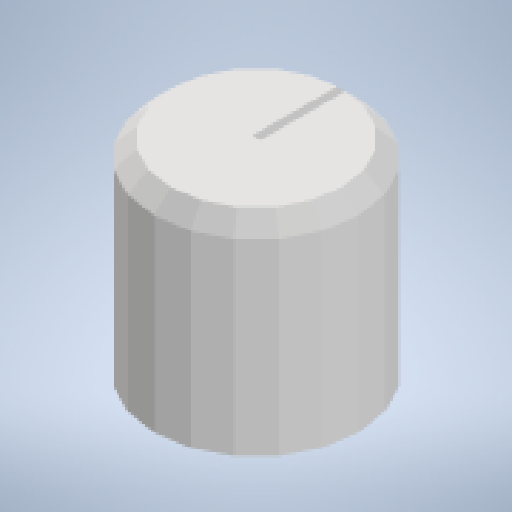
# Autodesk Inventor part: PotiBoxKnob
Saved by Autodesk Inventor 2024.3 (Build 283343000, 343)
## iProperties
Created: 2025-03-30
Part Number: PotiBoxKnob
Material: Generisch
Document SubType Name: Modeling
Designer: maxho
Density: 1 g/cm^3
Appearance: Vorgabe
Author: maxho
## iProperties of the stored document PotiBoxKnob_3D-Druck.ipt
Created: 2025-03-30
Part Number: PotiBoxKnob_3D-Druck
Material: Generisch
Document SubType Name: Modeling
Designer: maxho
Density: 1 g/cm^3
Appearance: Vorgabe
Author: maxho
Autodesk Inventor part; units mm, degrees
ref_plane "YZ Plane" through (0, 0, 0) normal (1, 0, 0) x (0, 1, 0)
ref_plane "XZ Plane" through (0, 0, 0) normal (0, 1, 0) x (-1, 0, 0)
ref_plane "XY Plane" through (0, 0, 0) normal (0, 0, 1) x (1, 0, 0)
sketch "Skizze1" plane through (0, 0, 0) normal (0, 0, 1) x (1, 0, 0)
  circle A0 centre (0, 0) radius 12.5 construction
  line L0 (-0.5, 16.5) -> (0.5, 16.5)
  line L1 (0.5, 16.5) -> (0.5, 11.5)
  line L2 (0.5, 11.5) -> (-0.5, 11.5)
  line L3 (-0.5, 11.5) -> (-0.5, 16.5)
  line L4 (0, -12.5) -> (-3.8627, -11.8882)
  line L5 (-3.8627, -11.8882) -> (-7.3473, -10.1127)
  line L6 (-7.3473, -10.1127) -> (-10.1127, -7.3473)
  line L7 (-10.1127, -7.3473) -> (-11.8882, -3.8627)
  line L8 (-11.8882, -3.8627) -> (-12.5, 0)
  line L9 (-12.5, 0) -> (-11.8882, 3.8627)
  line L10 (-11.8882, 3.8627) -> (-10.1127, 7.3473)
  line L11 (-10.1127, 7.3473) -> (-7.3473, 10.1127)
  line L12 (-7.3473, 10.1127) -> (-3.8627, 11.8882)
  line L13 (-3.8627, 11.8882) -> (0, 12.5)
  line L14 (0, 12.5) -> (3.8627, 11.8882)
  line L15 (3.8627, 11.8882) -> (7.3473, 10.1127)
  line L16 (7.3473, 10.1127) -> (10.1127, 7.3473)
  line L17 (10.1127, 7.3473) -> (11.8882, 3.8627)
  line L18 (11.8882, 3.8627) -> (12.5, 0)
  line L19 (12.5, 0) -> (11.8882, -3.8627)
  line L20 (11.8882, -3.8627) -> (10.1127, -7.3473)
  line L21 (10.1127, -7.3473) -> (7.3473, -10.1127)
  line L22 (7.3473, -10.1127) -> (3.8627, -11.8882)
  line L23 (3.8627, -11.8882) -> (0, -12.5)
  point P0 (0, 11.5)
  point P1 (-0.5, 12.49)
  point P2 (0.5, 12.49)
  point P3 (-0.5, 12.4208)
  point P4 (0.5, 12.4208)
  dimension "d0" = 25
  dimension "d3" = 1
  dimension "d4" = 1
  dimension "d12" = 5
  constraints: 48 end point, 2 coincident, 2 parallel, 2 vertical alignment, 1 horizontal, 1 midpoint, 1 perpendicular, 44 other
  measures "d3" length of L2
  measures "d4" distance of L0.start L0.end
  measures "d12" distance between parallel lines of L0 L2
extrude "Extrusion1" add sketch "Skizze1" along normal blind 25 contours L3 L2 L1 L14 L15 L16 L17 L18 L19 L20 L21 L22 L23 L4 L5 L6 L7 L8 L9 L10 L11 L12 L13
sketch "Skizze4" plane through (0, 0, 25) normal (0, 0, 1) x (1, 0, 0)
  line L0 (-0.5, 11.5) -> (-0.5, 12.4208) projected
  line L1 (-0.5, 12.4208) -> (-3.8627, 11.8882) projected
  line L2 (-3.8627, 11.8882) -> (-7.3473, 10.1127) projected
  line L3 (-7.3473, 10.1127) -> (-10.1127, 7.3473) projected
  line L4 (-10.1127, 7.3473) -> (-11.8882, 3.8627) projected
  line L5 (-11.8882, 3.8627) -> (-12.5, 0) projected
  line L6 (-12.5, 0) -> (-11.8882, -3.8627) projected
  line L7 (-11.8882, -3.8627) -> (-10.1127, -7.3473) projected
  line L8 (-10.1127, -7.3473) -> (-7.3473, -10.1127) projected
  line L9 (-7.3473, -10.1127) -> (-3.8627, -11.8882) projected
  line L10 (-3.8627, -11.8882) -> (0, -12.5) projected
  line L11 (0, -12.5) -> (3.8627, -11.8882) projected
  line L12 (3.8627, -11.8882) -> (7.3473, -10.1127) projected
  line L13 (7.3473, -10.1127) -> (10.1127, -7.3473) projected
  line L14 (10.1127, -7.3473) -> (11.8882, -3.8627) projected
  line L15 (11.8882, -3.8627) -> (12.5, 0) projected
  line L16 (12.5, 0) -> (11.8882, 3.8627) projected
  line L17 (11.8882, 3.8627) -> (10.1127, 7.3473) projected
  line L18 (10.1127, 7.3473) -> (7.3473, 10.1127) projected
  line L19 (7.3473, 10.1127) -> (3.8627, 11.8882) projected
  line L20 (3.8627, 11.8882) -> (0.5, 12.4208) projected
  line L21 (0.5, 12.4208) -> (0.5, 11.5) projected
  line L22 (0.5, 11.5) -> (-0.5, 11.5) projected
  line L23 (0.5, 11.5) -> (-0.5, 11.5)
  line L24 (-0.5, 11.5) -> (-0.5, 0)
  line L25 (-0.5, 0) -> (0.5, 0)
  line L26 (0.5, 0) -> (0.5, 11.5)
  point P0 (0, 0)
  constraints: 8 end point, 2 parallel, 1 horizontal, 1 midpoint, 1 perpendicular
extrude "Extrusion3" cut sketch "Skizze4" against normal blind 2 contours L22 L26 L25 L24
sketch "Skizze2" plane through (0, 0, 0) normal (0, 0, -1) x (-1, 0, 0)
  point P0 (0, 0)
  point P1 (0, 0)
  constraints: 1 coincident
hole "Bohrung1" at (0, 0, 0) direction (0, 0, 1) diameter 6.34 depth 20.62 counterbore diameter 20 counterbore depth 8.9375
sketch "Skizze3" plane through (0, 0, 20.62) normal (0, 0, -1) x (-1, 0, 0)
  line L0 (-3.17, 0.25) -> (3.17, 0.25)
  line L1 (3.17, 0.25) -> (3.17, -0.25)
  line L2 (3.17, -0.25) -> (-3.17, -0.25)
  line L3 (-3.17, -0.25) -> (-3.17, 0.25)
  line L4 (-3.17, 0.25) -> (3.17, -0.25) construction
  line L5 (3.17, 0.25) -> (-3.17, -0.25) construction
  circle A0 centre (0, 0) radius 3.17 projected
  circle A1 centre (0, 0) radius 3.17 projected
  point P0 (3.17, 0)
  dimension "d13" = 0.5
  constraints: 12 end point, 3 midpoint, 2 parallel, 1 horizontal, 1 horizontal alignment, 1 perpendicular, 1 other
  measures "d13" distance between parallel lines of L0 L2
extrude "Extrusion2" add sketch "Skizze3" along normal blind 0.5 contours L0 A0 L3 | L0 A0 L2 | A0 L2 L3 | L0 L1 A0 | L1 L2 A0
chamfer "Fasen1" distance 2 angle 45 21 edges at (11.0005, -5.605, 25) (12.1941, -1.9314, 25) (12.1941, 1.9314, 25) (11.0005, 5.605, 25) (8.73, 8.73, 25) (5.605, 11.0005, 25) (2.1814, 12.1545, 25) (-2.1814, 12.1545, 25) (-5.605, 11.0005, 25) (-8.73, 8.73, 25) (-11.0005, 5.605, 25) (-12.1941, 1.9314, 25) (-12.1941, -1.9314, 25) (-11.0005, -5.605, 25) (-8.73, -8.73, 25) (-5.605, -11.0005, 25) (-1.9314, -12.1941, 25) (1.9314, -12.1941, 25) (5.605, -11.0005, 25) (8.73, -8.73, 25) (0, 11.5, 23)
equation "\"d0\" = KnobDiameter"
equation "\"d1\" = KnobHeight"
equation "\"d5\" = PotiShaftDiameter"
equation "\"KnobDiameter\" = 25"
equation "\"KnobHeight\" = 25"
equation "\"PotiShaftDiameter\" = 6.34"
